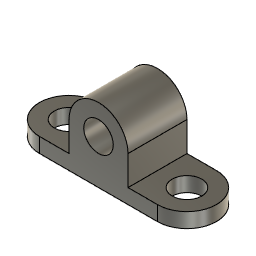
A4 (Autodesk Fusion 360 design; units mm, degrees)
Autodesk Fusion 360 part; units mm, degrees
sketch "base" plane through (0, 0, 0) normal (0, 0, 1) x (1, 0, 0)
  line L0 (60, 20) -> (-60, 20)
  line L1 (-60, 20) -> (-60, -20)
  line L2 (-60, -20) -> (60, -20)
  line L3 (60, -20) -> (60, 20)
  line L4 (60, 20) -> (-60, -20) construction
  line L5 (-60, 20) -> (60, -20) construction
  dimension "d1" = 120
  dimension "d2" = 40
  constraint horizontal L0
  constraint perpendicular L0 L1
  constraint parallel L0 L2
  constraint parallel L1 L3
  constraint coincident L4 origin
  constraint coincident L5 origin
  measures "d1" distance of L1.end L2.end
  measures "d2" distance of L0.end L1.end
extrude "Extrude1" add sketch "base" along normal blind 10
fillet "Fillet1" radius 20 4 edges at (60, -20, 5) (-60, -20, 5) (60, 20, 5) (-60, 20, 5)
sketch "center square" plane through (0, 0, 10) normal (0, 0, 1) x (-1, 0, 0)
  arc A0 (40, -20) -> (40, 20) centre (40, 0) ccw
  line L0 (40, 20) -> (-40, 20)
  arc A1 (-40, 20) -> (-40, -20) centre (-40, 0) ccw
  line L1 (-40, -20) -> (40, -20)
  line L2 (20, 20) -> (-20, 20)
  line L3 (-20, 20) -> (-20, -20)
  line L4 (-20, -20) -> (20, -20)
  line L5 (20, -20) -> (20, 20)
  dimension "d6" = 20
  dimension "d7" = 40
  dimension "d8" = 40
  constraint horizontal L2
  constraint vertical L3
  constraint horizontal L4
  constraint vertical L5
  measures "d6" distance of A0.end L2.start
  measures "d7" distance of L2.start L2.end
  measures "d8" distance of L2.start L4.end
extrude "Extrude2" add sketch "center square" along normal blind 40 contours L0 L1 L2 L3 L4 L5
fillet "Fillet2" radius 20 2 edges at (-20, 0, 50) (20, 0, 50)
sketch "left circle" plane through (0, 0, 10) normal (0, 0, 1) x (-1, 0, 0)
  line L0 (20, 20) -> (20, -20)
  line L1 (20, -20) -> (40, -20)
  arc A0 (40, -20) -> (40, 20) centre (40, 0) ccw
  line L2 (40, 20) -> (20, 20)
  line L3 (40, 20) -> (40, -20) construction
  circle A1 centre (40, 0) radius 10
  dimension "d12" = 20
  constraint coincident A0.end L2.start
  constraint coincident L1.end A0.start
  constraint concentric A0 A1
  measures "d12" diameter of A1
sketch "right circle" plane through (0, 0, 10) normal (0, 0, 1) x (-1, 0, 0)
  line L0 (-20, -20) -> (-20, 20)
  line L1 (-20, 20) -> (-40, 20)
  arc A0 (-40, 20) -> (-40, -20) centre (-40, 0) ccw
  line L2 (-40, -20) -> (-20, -20)
  line L3 (-40, 20) -> (-40, -20) construction
  circle A1 centre (-40, 0) radius 10
  dimension "d13" = 20
  constraint coincident L1.end A0.start
  constraint coincident A0.end L2.start
  constraint concentric A0 A1
  measures "d13" diameter of A1
extrude "Extrude3" cut sketch "right circle" sketch "left circle" against normal blind 48 contours A1 of sketch 2 contours A1
sketch "front circle" plane through (0, -20, 0) normal (0, -1, 0) x (1, 0, 0)
  arc A0 (20, 30) -> (-20, 30) centre (0, 30) ccw
  line L0 (-20, 30) -> (-20, 10)
  line L1 (-20, 10) -> (-40, 10)
  line L2 (-40, 10) -> (-40, 0)
  line L3 (-40, 0) -> (40, 0)
  line L4 (40, 0) -> (40, 10)
  line L5 (40, 10) -> (20, 10)
  line L6 (20, 10) -> (20, 30)
  line L7 (-20, 30) -> (20, 30) construction
  circle A1 centre (0, 30) radius 10
  dimension "d16" = 20
  constraint coincident A0.end L0.start
  constraint coincident A0.start L6.end
  constraint concentric A0 A1
  measures "d16" diameter of A1
extrude "Extrude4" cut sketch "front circle" against normal blind 62 contours A1
equation "d1 = 20 mm + 20 mm + 40 mm + 20 mm + 20 mm"
named bodies: "A4"
